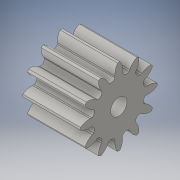
# Autodesk Inventor part: Alligator_Pinion (2)
Saved by Autodesk Inventor 2016 (Build 200138000, 138)
## iProperties
Created: 2017-05-22
Part Number: Alligator_Pinion (2)
Material: Generic
Document SubType Name: Modeling
Designer: nazardio000
Density: 1 g/cm^3
Appearance: Default
Author: nazardio000
Autodesk Inventor part; units mm, degrees
ref_plane "YZ Plane" through (0, 0, 0) normal (1, 0, 0) x (0, 1, 0)
ref_plane "XZ Plane" through (0, 0, 0) normal (0, 1, 0) x (-1, 0, 0)
ref_plane "Work Plane2" through (2.8575, 0, 0) normal (1, 0, 0) x (0, 0, -1)
sketch "Sketch6" plane through (2.8575, 0, 0) normal (1, 0, 0) x (0, 0, -1)
  line L0 (0.7654, -5.6784) -> (0.7654, -5.022)
  line L1 (-0.7638, -5.6784) -> (-0.7638, -5.0222)
  arc A0 (5.6006, 2.3498) -> (5.5837, 2.3418) centre (6.3532, 0.7382) ccw
  arc A1 (-0.7638, -5.0222) -> (0.7654, -5.022) centre (0, 0) ccw
  line L2 (0.0008, -7.62) -> (-0.2439, -7.62)
  line L3 (0.0008, -7.62) -> (0.2479, -7.62)
  arc A2 (0.2479, -7.62) -> (0.7654, -5.6784) centre (-2.309, -5.8988) ccw
  arc A3 (-0.7638, -5.6784) -> (-0.2439, -7.62) centre (2.2185, -5.9201) ccw
  arc A4 (3.5877, -3.5965) -> (3.5976, -3.5866) centre (0, 0) ccw
  line L4 (3.502, -4.5349) -> (3.1738, -3.9665)
  line L5 (2.1777, -5.2996) -> (1.8496, -4.7313)
  arc A5 (1.8496, -4.7313) -> (3.1738, -3.9665) centre (0, 0) ccw
  line L6 (3.8107, -6.5987) -> (3.5988, -6.721)
  line L7 (3.8107, -6.5987) -> (4.0247, -6.4752)
  arc A6 (4.0247, -6.4752) -> (3.502, -4.5349) centre (0.9498, -6.263) ccw
  arc A7 (2.1777, -5.2996) -> (3.5988, -6.721) centre (4.8813, -4.0177) ccw
  line L8 (5.3003, -2.1764) -> (4.7319, -1.8482)
  line L9 (4.5358, -3.5007) -> (3.9675, -3.1726)
  arc A8 (3.9675, -3.1726) -> (4.7319, -1.8482) centre (0, 0) ccw
  line L10 (6.5995, -3.8093) -> (6.4772, -4.0212)
  line L11 (6.5995, -3.8093) -> (6.7231, -3.5953)
  arc A9 (6.7231, -3.5953) -> (5.3003, -2.1764) centre (3.954, -4.949) ccw
  arc A10 (4.5358, -3.5007) -> (6.4772, -4.0212) centre (6.2362, -1.0388) ccw
  line L12 (5.6784, 0.7654) -> (5.022, 0.7654)
  line L13 (5.6784, -0.7638) -> (5.0222, -0.7638)
  arc A11 (5.0222, -0.7638) -> (5.022, 0.7654) centre (0, 0) ccw
  line L14 (7.62, 0.0008) -> (7.62, -0.2439)
  line L15 (7.62, 0.0008) -> (7.62, 0.2479)
  arc A12 (7.62, 0.2479) -> (5.6784, 0.7654) centre (5.8988, -2.309) ccw
  arc A13 (5.6784, -0.7638) -> (7.62, -0.2439) centre (5.9201, 2.2185) ccw
  line L16 (4.5349, 3.502) -> (3.9665, 3.1738)
  line L17 (5.2996, 2.1777) -> (4.7313, 1.8496)
  arc A14 (4.7313, 1.8496) -> (3.9665, 3.1738) centre (0, 0) ccw
  line L18 (6.5987, 3.8107) -> (6.721, 3.5988)
  line L19 (6.5987, 3.8107) -> (6.4752, 4.0247)
  arc A15 (6.4752, 4.0247) -> (4.5349, 3.502) centre (6.263, 0.9498) ccw
  arc A16 (5.2996, 2.1777) -> (6.721, 3.5988) centre (4.0177, 4.8813) ccw
  line L20 (2.1764, 5.3003) -> (1.8482, 4.7319)
  line L21 (3.5007, 4.5358) -> (3.1726, 3.9675)
  arc A17 (3.1726, 3.9675) -> (1.8482, 4.7319) centre (0, 0) ccw
  line L22 (3.8093, 6.5995) -> (4.0212, 6.4772)
  line L23 (3.8093, 6.5995) -> (3.5953, 6.7231)
  arc A18 (3.5953, 6.7231) -> (2.1764, 5.3003) centre (4.949, 3.954) ccw
  arc A19 (3.5007, 4.5358) -> (4.0212, 6.4772) centre (1.0388, 6.2362) ccw
  line L24 (-0.7654, 5.6784) -> (-0.7654, 5.022)
  line L25 (0.7638, 5.6784) -> (0.7638, 5.0222)
  arc A20 (0.7638, 5.0222) -> (-0.7654, 5.022) centre (0, 0) ccw
  line L26 (-0.0008, 7.62) -> (0.2439, 7.62)
  line L27 (-0.0008, 7.62) -> (-0.2479, 7.62)
  arc A21 (-0.2479, 7.62) -> (-0.7654, 5.6784) centre (2.309, 5.8988) ccw
  arc A22 (0.7638, 5.6784) -> (0.2439, 7.62) centre (-2.2185, 5.9201) ccw
  line L28 (-3.502, 4.5349) -> (-3.1738, 3.9665)
  line L29 (-2.1777, 5.2996) -> (-1.8496, 4.7313)
  arc A23 (-1.8496, 4.7313) -> (-3.1738, 3.9665) centre (0, 0) ccw
  line L30 (-3.8107, 6.5987) -> (-3.5988, 6.721)
  line L31 (-3.8107, 6.5987) -> (-4.0247, 6.4752)
  arc A24 (-4.0247, 6.4752) -> (-3.502, 4.5349) centre (-0.9498, 6.263) ccw
  arc A25 (-2.1777, 5.2996) -> (-3.5988, 6.721) centre (-4.8813, 4.0177) ccw
  line L32 (-5.3003, 2.1764) -> (-4.7319, 1.8482)
  line L33 (-4.5358, 3.5007) -> (-3.9675, 3.1726)
  arc A26 (-3.9675, 3.1726) -> (-4.7319, 1.8482) centre (0, 0) ccw
  line L34 (-6.5995, 3.8093) -> (-6.4772, 4.0212)
  line L35 (-6.5995, 3.8093) -> (-6.7231, 3.5953)
  arc A27 (-6.7231, 3.5953) -> (-5.3003, 2.1764) centre (-3.954, 4.949) ccw
  arc A28 (-4.5358, 3.5007) -> (-6.4772, 4.0212) centre (-6.2362, 1.0388) ccw
  line L36 (-5.6784, -0.7654) -> (-5.022, -0.7654)
  line L37 (-5.6784, 0.7638) -> (-5.0222, 0.7638)
  arc A29 (-5.0222, 0.7638) -> (-5.022, -0.7654) centre (0, 0) ccw
  line L38 (-7.62, -0.0008) -> (-7.62, 0.2439)
  line L39 (-7.62, -0.0008) -> (-7.62, -0.2479)
  arc A30 (-7.62, -0.2479) -> (-5.6784, -0.7654) centre (-5.8988, 2.309) ccw
  arc A31 (-5.6784, 0.7638) -> (-7.62, 0.2439) centre (-5.9201, -2.2185) ccw
  line L40 (-4.5349, -3.502) -> (-3.9665, -3.1738)
  line L41 (-5.2996, -2.1777) -> (-4.7313, -1.8496)
  arc A32 (-4.7313, -1.8496) -> (-3.9665, -3.1738) centre (0, 0) ccw
  line L42 (-6.5987, -3.8107) -> (-6.721, -3.5988)
  line L43 (-6.5987, -3.8107) -> (-6.4752, -4.0247)
  arc A33 (-6.4752, -4.0247) -> (-4.5349, -3.502) centre (-6.263, -0.9498) ccw
  arc A34 (-5.2996, -2.1777) -> (-6.721, -3.5988) centre (-4.0177, -4.8813) ccw
  line L44 (-2.1764, -5.3003) -> (-1.8482, -4.7319)
  line L45 (-3.5007, -4.5358) -> (-3.1726, -3.9675)
  arc A35 (-3.1726, -3.9675) -> (-1.8482, -4.7319) centre (0, 0) ccw
  line L46 (-3.8093, -6.5995) -> (-4.0212, -6.4772)
  line L47 (-3.8093, -6.5995) -> (-3.5953, -6.7231)
  arc A36 (-3.5953, -6.7231) -> (-2.1764, -5.3003) centre (-4.949, -3.954) ccw
  arc A37 (-3.5007, -4.5358) -> (-4.0212, -6.4772) centre (-1.0388, -6.2362) ccw
  arc A38 (-1.8482, -4.7319) -> (-0.7638, -5.0222) centre (0, 0) ccw
  line L48 (-2.0137, 5.0155) -> (-0.7654, 5.3502)
  line L49 (0.7638, 5.3503) -> (2.0123, 5.0161)
  line L50 (3.3367, 4.2516) -> (4.2507, 3.3379)
  line L51 (5.0155, 2.0137) -> (5.3502, 0.7654)
  line L52 (5.3503, -0.7638) -> (5.0161, -2.0123)
  line L53 (4.2516, -3.3367) -> (3.3379, -4.2507)
  line L54 (2.0137, -5.0155) -> (0.7654, -5.3502)
  line L55 (-0.7638, -5.3503) -> (-2.0123, -5.0161)
  line L56 (-3.3367, -4.2516) -> (-4.2507, -3.3379)
  line L57 (-5.0155, -2.0137) -> (-5.3502, -0.7654)
  line L58 (-5.3503, 0.7638) -> (-5.0161, 2.0123)
  line L59 (-4.2516, 3.3367) -> (-3.3379, 4.2507)
  circle A39 centre (0, 0) radius 5.0531
  point P0 (0, 0)
  point P1 (-4.2516, 3.3367)
  dimension "d94" = 360
  constraints: 120 end point, 78 point on circle, 40 centre point, 9 perpendicular, 3 midpoint, 2 horizontal, 1 coincident, 1 parallel, 1 vertical, 229 other
extrude "Extrusion19" add sketch "Sketch6" against normal blind 11.4554 contours A2 L3 L2 A3 L1 A1 L0 | L0 A1 A38 A35 L45 L56 L40 A32 L41 L57 L36 A29 L37 L58 L32 A26 L33 L59 L28 A23 L29 L48 L24 A20 L25 L49 L20 A17 L21 L50 L16 A14 L17 L51 L12 A11 L13 L52 L8 A8 L9 L53 L4 A5 L5 L54 | L5 A5 L4 A6 L7 L6 A7 | L1 L55 L44 A38 | L44 A36 L47 L46 A37 L45 A35 | L9 A8 L8 A9 L11 L10 A10 | L40 A33 L43 L42 A34 L41 A32 | L13 A11 L12 A12 L15 L14 A13 | L36 A30 L39 L38 A31 L37 A29 | L17 A14 L16 A15 L19 L18 A16 | L32 A27 L35 L34 A28 L33 A26 | L21 A17 L20 A18 L23 L22 A19 | L28 A24 L31 L30 A25 L29 A23 | L25 A20 L24 A21 L27 L26 A22 | A39
sketch "Sketch7" plane through (-8.5979, 0, 0) normal (-1, 0, 0) x (0, 0, 1)
  circle A0 centre (0, 0) radius 1.625
  dimension "d104" = 3.25
  constraints: 1 centre point, 1 coincident
  measures "d104" diameter of A0
extrude "Extrusion20" cut sketch "Sketch7" against normal blind 2540
sketch "Sketch8" plane through (-8.5979, 0, 0) normal (-1, 0, 0) x (0, 0, 1)
  circle A0 centre (0, 0) radius 5.08
  line L0 (-3.3367, 4.2516) -> (-4.2507, 3.3379) projected
  arc A1 (-4.2507, 3.3379) -> (-3.3367, 4.2516) centre (-4.209, 4.2103) ccw
  line L1 (-3.3367, 4.2516) -> (-3.5007, 4.5358) projected
  line L2 (-4.2507, 3.3379) -> (-3.3367, 4.2516)
  arc A2 (-5.3502, 0.7654) -> (-5.0155, 2.0137) centre (-5.7503, 1.5417) ccw
  line L3 (-5.3502, 0.7654) -> (-5.0155, 2.0137)
  arc A3 (-5.0161, -2.0123) -> (-5.3503, -0.7638) centre (-5.7507, -1.54) ccw
  line L4 (-5.0161, -2.0123) -> (-5.3503, -0.7638)
  arc A4 (-3.3379, -4.2507) -> (-4.2516, -3.3367) centre (-4.2103, -4.209) ccw
  line L5 (-3.3379, -4.2507) -> (-4.2516, -3.3367)
  arc A5 (-0.7654, -5.3502) -> (-2.0137, -5.0155) centre (-1.5417, -5.7503) ccw
  line L6 (-0.7654, -5.3502) -> (-2.0137, -5.0155)
  arc A6 (2.0123, -5.0161) -> (0.7638, -5.3503) centre (1.54, -5.7507) ccw
  line L7 (2.0123, -5.0161) -> (0.7638, -5.3503)
  arc A7 (4.2507, -3.3379) -> (3.3367, -4.2516) centre (4.209, -4.2103) ccw
  line L8 (4.2507, -3.3379) -> (3.3367, -4.2516)
  arc A8 (5.3502, -0.7654) -> (5.0155, -2.0137) centre (5.7503, -1.5417) ccw
  line L9 (5.3502, -0.7654) -> (5.0155, -2.0137)
  arc A9 (5.0161, 2.0123) -> (5.3503, 0.7638) centre (5.7507, 1.54) ccw
  line L10 (5.0161, 2.0123) -> (5.3503, 0.7638)
  arc A10 (3.3379, 4.2507) -> (4.2516, 3.3367) centre (4.2103, 4.209) ccw
  line L11 (3.3379, 4.2507) -> (4.2516, 3.3367)
  arc A11 (0.7654, 5.3502) -> (2.0137, 5.0155) centre (1.5417, 5.7503) ccw
  line L12 (0.7654, 5.3502) -> (2.0137, 5.0155)
  arc A12 (-2.0123, 5.0161) -> (-0.7638, 5.3503) centre (-1.54, 5.7507) ccw
  line L13 (-2.0123, 5.0161) -> (-0.7638, 5.3503)
  dimension "d107" = 10.16
  dimension "d110" = 360
  constraints: 24 end point, 24 point on circle, 13 centre point, 1 coincident, 1 tangent, 61 other
  measures "d107" diameter of A0
extrude "Extrusion21" cut sketch "Sketch8" against normal blind 2540 contours A8 L9 | A7 L8 | A6 L7 | A5 L6 | A4 L5 | A3 L4 | A2 L3 | A1 L0 | A12 L13 | A11 L12 | A10 L11 | A9 L10
body "Solid1"
